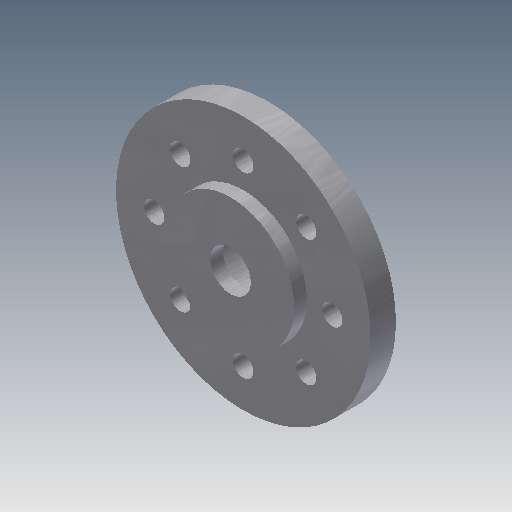
# Autodesk Inventor part: アルミローハイトサーボホーン
Saved by Autodesk Inventor 2019.4 (Build 234330000, 330)
## iProperties
Created: 2014-02-23
Part Number: アルミローハイトサーボホーン
Material: アルミニウム 2014-T4
Document SubType Name: Modeling
Designer: HKenta
Density: 2.8 g/cm^3
Appearance: サテン
Mass: 1.84902 g
Surface Area: 9.15586 cm^2
Volume: 0.660363 cm^3
Author: HKenta
Autodesk Inventor part; units mm, degrees
ref_plane "YZ Plane" through (0, 0, 0) normal (1, 0, 0) x (0, 1, 0)
ref_plane "XZ Plane" through (0, 0, 0) normal (0, 1, 0) x (-1, 0, 0)
ref_plane "XY Plane" through (0, 0, 0) normal (0, 0, 1) x (1, 0, 0)
sketch "スケッチ1" plane through (0, 0, 0) normal (0, 0, 1) x (1, 0, 0)
  circle A0 centre (0, 0) radius 10
  circle A1 centre (0, 0) radius 1.6
  circle A2 centre (0, 0) radius 7 construction
  circle A3 centre (0, 7) radius 0.8
  line L0 (0, 7) -> (0, 0) construction
  circle A4 centre (-4.9497, 4.9497) radius 0.8
  circle A5 centre (-7, 0) radius 0.8
  circle A6 centre (-4.9497, -4.9497) radius 0.8
  circle A7 centre (0, -7) radius 0.8
  circle A8 centre (4.9497, -4.9497) radius 0.8
  circle A9 centre (7, 0) radius 0.8
  circle A10 centre (4.9497, 4.9497) radius 0.8
  dimension "d2" = 14
  dimension "d0" = 20
  dimension "d1" = 3.2
  dimension "d3" = 1.6
  dimension "d6" = 360
  constraints: 10 centre point, 3 coincident, 2 end point, 1 vertical, 1 vertical alignment, 19 other
  measures "d0" diameter of A0
  measures "d1" diameter of A1
  measures "d3" diameter of A3
extrude "押し出し1" add sketch "スケッチ1" along normal blind 2
sketch "スケッチ2" plane through (0, 0, 2) normal (0, 0, 1) x (1, 0, 0)
  circle A0 centre (0, 0) radius 1.6 projected
  circle A1 centre (0, 0) radius 10 projected
  circle A2 centre (0, 0) radius 5
  dimension "d10" = 10
  constraints: 1 centre point, 1 coincident
  measures "d10" diameter of A2
extrude "押し出し2" add sketch "スケッチ2" along normal blind 1 contours A2
sketch "スケッチ3" plane through (0, 0, 0) normal (0, 0, -1) x (-1, 0, 0)
  circle A0 centre (0, 0) radius 1.6 projected
  circle A1 centre (0, 0) radius 10 projected
  circle A2 centre (0, 0) radius 5
  dimension "d13" = 10
  constraints: 1 centre point, 1 coincident
  measures "d13" diameter of A2
extrude "押し出し3" add sketch "スケッチ3" along normal blind 1 contours A2
sketch "スケッチ4" plane through (0, 0, -1) normal (0, 0, -1) x (-1, 0, 0)
  circle A0 centre (0, 0) radius 1.6 projected
  circle A1 centre (0, 0) radius 5 projected
  circle A2 centre (0, 0) radius 3
  dimension "d16" = 6
  constraints: 1 centre point, 1 coincident
  measures "d16" diameter of A2
extrude "押し出し4" cut sketch "スケッチ4" against normal blind 3 contours A2
